Autodesk Fusion 360 part; units mm, degrees
note: some values were not read from the file. Set by a fixed rule: which sketch regions a step uses.
(part 3 of 3)
  line L1807 (17.4645, -45.5732) -> (17.4645, -44.8732)
  line L1808 (18.1645, -45.5732) -> (17.4645, -45.5732)
  line L1809 (18.1645, -44.8732) -> (18.1645, -45.5732)
  line L1810 (17.4645, -47.4132) -> (18.1645, -47.4132)
  line L1811 (17.4645, -48.1132) -> (17.4645, -47.4132)
  line L1812 (18.1645, -48.1132) -> (17.4645, -48.1132)
  line L1813 (18.1645, -47.4132) -> (18.1645, -48.1132)
  line L1814 (17.4645, -49.9532) -> (18.1645, -49.9532)
  line L1815 (17.4645, -50.6532) -> (17.4645, -49.9532)
  line L1816 (18.1645, -50.6532) -> (17.4645, -50.6532)
  line L1817 (18.1645, -49.9532) -> (18.1645, -50.6532)
  line L1818 (51.7545, -37.9058) -> (51.7545, -37.2058)
  line L1819 (51.7545, -37.2058) -> (52.4545, -37.2058)
  line L1820 (52.4545, -37.9058) -> (51.7545, -37.9058)
  line L1821 (52.4545, -37.2058) -> (52.4545, -37.9058)
  line L1822 (51.7545, -40.4458) -> (51.7545, -39.7458)
  line L1823 (51.7545, -39.7458) -> (52.4545, -39.7458)
  line L1824 (52.4545, -40.4458) -> (51.7545, -40.4458)
  line L1825 (52.4545, -39.7458) -> (52.4545, -40.4458)
  line L1826 (51.7545, -42.9858) -> (51.7545, -42.2858)
  line L1827 (51.7545, -42.2858) -> (52.4545, -42.2858)
  line L1828 (52.4545, -42.9858) -> (51.7545, -42.9858)
  line L1829 (52.4545, -42.2858) -> (52.4545, -42.9858)
  line L1830 (51.7545, -45.5258) -> (51.7545, -44.8258)
  line L1831 (51.7545, -44.8258) -> (52.4545, -44.8258)
  line L1832 (52.4545, -45.5258) -> (51.7545, -45.5258)
  line L1833 (52.4545, -44.8258) -> (52.4545, -45.5258)
  line L1834 (51.7545, -48.0658) -> (51.7545, -47.3658)
  line L1835 (51.7545, -47.3658) -> (52.4545, -47.3658)
  line L1836 (52.4545, -48.0658) -> (51.7545, -48.0658)
  line L1837 (52.4545, -47.3658) -> (52.4545, -48.0658)
  line L1838 (51.7545, -50.6058) -> (51.7545, -49.9058)
  line L1839 (51.7545, -49.9058) -> (52.4545, -49.9058)
  line L1840 (52.4545, -50.6058) -> (51.7545, -50.6058)
  line L1841 (52.4545, -49.9058) -> (52.4545, -50.6058)
  line L1842 (11.4445, -17.8682) -> (16.7445, -28.1482)
  line L1843 (11.4445, -28.1482) -> (16.7445, -17.8682)
  line L1844 (18.0945, -17.8682) -> (10.0945, -17.8682)
  line L1845 (10.0945, -17.8682) -> (10.0945, -28.1482)
  line L1846 (10.0945, -28.1482) -> (18.0945, -28.1482)
  line L1847 (18.0945, -28.1482) -> (18.0945, -17.8682)
  line L1848 (18.0945, -17.8682) -> (10.0945, -28.1482) construction
  line L1849 (10.0945, -17.8682) -> (18.0945, -28.1482) construction
  point P0 (62.6345, -26.9982)
  point P1 (68.3345, -18.4982)
  point P2 (5.5845, -52.2482)
  point P3 (68.3345, -52.2482)
  point P4 (4.8345, -21.9982)
  point P5 (52.1045, -35.0158)
  point P6 (17.8145, -31.4432)
  point P7 (17.8145, -40.1432)
  point P8 (14.0945, -23.0082)
  dimension "d3" = 0.7
  dimension "d4" = 0.7
  dimension "d5" = 0.7
  dimension "d6" = 0.7
  dimension "d7" = 0.7
  dimension "d8" = 0.7
  dimension "d11" = 5.08
  dimension "d12" = 0
  dimension "d15" = 10.16
  dimension "d16" = 0
  dimension "d19" = 15.24
  dimension "d20" = 0
  dimension "d21" = 8
  text T0 "+" font "Arial" height 1.3333 align ink ink in box 0 x 0 at (53.2945, -25.6783) x (1, 0) y (0, 1) spacing 1 height is em
  constraint horizontal L1746
  constraint vertical L1747
  constraint horizontal L1748
  constraint vertical L1749
  constraint horizontal L1750
  constraint vertical L1751
  constraint horizontal L1752
  constraint vertical L1753
  constraint horizontal L1754
  constraint vertical L1755
  constraint horizontal L1756
  constraint vertical L1757
  constraint horizontal L1758
  constraint vertical L1759
  constraint horizontal L1760
  constraint vertical L1761
  constraint horizontal L1762
  constraint vertical L1763
  constraint horizontal L1764
  constraint vertical L1765
  constraint horizontal L1766
  constraint vertical L1767
  constraint horizontal L1768
  constraint vertical L1769
  constraint horizontal L1776
  constraint perpendicular L1776 L1777
  constraint parallel L1776 L1778
  constraint parallel L1777 L1779
  constraint coincident L1780 P5
  constraint coincident L1781 P5
  constraint midpoint L1774 P5
  constraint horizontal L1782
  constraint perpendicular L1782 L1783
  constraint parallel L1782 L1784
  constraint parallel L1783 L1785
  constraint coincident L1786 P6
  constraint coincident L1787 P6
  constraint midpoint L1770 P6
  constraint horizontal L1788
  constraint perpendicular L1788 L1789
  constraint parallel L1788 L1790
  constraint parallel L1789 L1791
  constraint coincident L1792 P7
  constraint coincident L1793 P7
  constraint midpoint L1773 P7
  constraint horizontal L1844
  constraint perpendicular L1844 L1845
  constraint parallel L1844 L1846
  constraint parallel L1845 L1847
  constraint coincident L1848 P8
  constraint coincident L1849 P8
  constraint midpoint L1842 P8
  measures "d3" distance of L1777.end L1778.end
  measures "d4" distance of L1776.end L1777.end
  measures "d5" distance of L1783.end L1784.end
  measures "d6" distance of L1782.end L1783.end
  measures "d7" distance of L1789.end L1790.end
  measures "d8" distance of L1788.end L1789.end
  measures "d21" distance of L1845.end L1846.end
extrude "Extrude1" add sketch "Sketch1" sketch "Sketch1" against normal blind 1.6 contours L19 L20 L21 L22 L23 L24 L25 L26 L27 L28 L29 L30 | L70 L71 L74 | L72 L73 L74 | L94 L95 L96 L97 L98 L99 L100 L101 | L102 L103 L104 | L108 L113 L114 L115 L116 L117 L118 L119 L120 L121 | L157 L158 L159 | L155 L156 L159 | L162 L163 L164 | L160 L161 L164 | L169 L174 L175 L176 L177 L178 L179 L180 L181 L182 | L184 L185 L188 | L186 L187 L188 | L196 L197 L198 L199 L200 L201 L202 L203 L204 L205 | L229 L230 L231 L232 L233 L234 L235 L236 L237 L238 | L221 L222 L223 L224 L225 L226 L227 L228 L229 L238 | L246 L247 L248 L249 L250 L251 L252 L253 L254 L255 L256 L257 L258 L259 L260 L261 | L274 L275 L276 L277 L278 L279 L280 L281 L282 L283 | L321 L322 L323 L324 L325 L326 L327 L328 L329 L330 L331 L332 | L349 L350 L351 L352 L353 L354 L355 L356 L357 L358 | L442 L443 L444 L445 L446 L447 L448 L449 L450 L451 L452 L453 | L454 L455 L456 L457 L458 L459 L460 L461 L462 L463 L464 L465 | L521 L522 L523 L524 L525 L526 L527 L528 L529 L530 L531 L532 | L570 L571 L572 L573 L574 L575 L576 L577 L578 L579 L580 L581 | L658 L659 L660 L661 L662 L663 L664 L665 L666 L667 | L650 L651 L652 L653 L654 L655 L656 L657 L658 L667 | L706 L707 L708 | L704 L705 L708 | L716 L717 L718 L719 L720 L721 L722 L723 L724 L725 L726 L727 L728 L729 L730 L731 | L732 L733 L734 L735 L736 L737 L738 L739 L740 L741 L742 L743 L744 L745 L746 L747 | L747 L748 L749 L750 L751 L752 L753 L754 L755 L756 L757 L758 L759 L760 L761 L762 | L780 L781 L782 L783 L784 L785 L786 L787 L788 L789 L1570 L1575 L1576 | L779 L780 L789 L1565 L1566 L1567 L1568 L1569 L1570 | L772 L773 L774 L775 L776 L777 L778 L779 L1565 L1566 L1567 L1568 L1569 L1570 | L781 L782 L1575 L1576 | L791 L792 L1573 L1574 | L791 L792 L1573 | L792 L1573 L1574 | L801 L802 L803 L804 L805 L806 L807 L808 A1 | L801 L802 L803 L804 L805 L806 L807 L808 A1 L1844 | L1654 L1655 L1842 L1843 L1844 | L1652 L1842 L1843 | L1652 L1844 L1845 L1846 | L1653 L1842 L1843 L1846 | L1656 L1842 L1843 | L1656 L1844 L1846 L1847 | L819 L820 L821 L822 L823 L824 L825 L826 L827 L828 L829 L830 | L868 L869 L870 L871 L872 L873 L874 L875 L876 L877 L878 L879 L880 L881 L882 L883 L884 L885 L886 L887 | L926 L927 L928 L929 L930 L931 L932 L933 L934 L935 | L918 L919 L920 L921 L922 L923 L924 L925 L926 L935 | L949 L950 L951 L952 L953 L954 L955 L956 L957 L958 L959 L960 L961 L962 L963 L964 | L1024 L1025 L1026 L1027 L1028 L1029 L1030 L1031 L1032 L1033 L1034 L1035 | L1037 L1038 L1039 L1040 L1041 L1042 L1043 L1044 L1045 L1046 L1047 L1048 L1049 L1050 L1051 L1052 | L1104 L1105 L1106 L1107 L1108 L1109 L1110 L1111 L1112 L1113 | L1096 L1097 L1098 L1099 L1100 L1101 L1102 L1103 L1104 L1113 | L1137 L1138 L1139 L1140 L1141 L1142 L1143 L1144 L1145 L1146 | L1157 L1158 L1159 L1160 L1161 L1162 L1163 L1164 L1165 L1166 L1167 L1168 L1169 L1170 L1171 L1172 L1173 L1174 L1175 L1176 | L1216 L1217 L1218 L1219 L1220 L1221 L1222 L1223 L1224 L1225 L1226 L1227 L1228 L1229 L1230 L1231 | L1233 L1234 L1237 | L1235 L1236 L1237 | L1265 L1266 L1267 L1268 L1269 L1270 L1271 L1272 | L1335 L1336 L1337 L1338 L1339 L1340 L1341 L1342 L1343 L1344 | L1327 L1328 L1329 L1330 L1331 L1332 L1333 L1334 L1335 L1344 | L1360 L1361 L1362 L1363 L1364 L1365 L1366 L1367 L1368 L1369 L1370 L1371 L1372 L1373 L1374 L1375 | L1412 L1413 L1414 L1415 L1416 L1417 L1418 L1419 L1420 L1421 L1422 L1423 L1424 L1425 L1426 L1427 | L1428 L1429 L1430 L1431 L1432 L1433 L1434 L1435 L1436 L1437 L1438 L1439 L1440 L1441 L1442 L1443 L1444 L1445 L1446 L1447 | L1500 L1501 L1502 L1503 L1504 L1505 L1506 L1507 L1508 L1509 L1510 L1511 L1512 L1513 L1514 L1515 | L1522 L1523 L1524 L1525 L1526 L1527 L1528 L1529 L1530 L1531 L1532 L1533 | L1539 L1540 L1541 L1542 L1543 L1544 L1545 L1546 L1547 L1548 L1549 L1550 L1551 L1552 L1553 L1554 | L1596 L1597 L1598 L1599 L1600 L1601 L1602 L1603 L1604 L1605 L1606 L1607 L1608 L1609 L1610 L1611 | L1612 L1613 L1614 L1615 L1616 L1617 L1618 L1619 L1620 L1621 L1622 L1623 L1624 L1625 L1626 L1627 L1628 L1629 L1630 L1631 | L1635 L1636 L1637 L1638 L1642 L1643 L1746 L1747 L1748 L1749 | L1639 L1640 L1641 | L1644 L1645 L1650 L1651 | A0 | L1658 L1761 L1772 L1773 L1789 | L1657 L1758 L1772 L1773 L1789 L1790 L1791 | L1772 L1773 L1789 L1790 L1791 | L1772 L1773 L1789 | L1759 L1772 L1773 L1791 | L1659 L1660 L1661 L1662 L1759 L1760 L1761 | L1660 L1772 L1773 L1788 L1789 L1791 | L1772 L1773 L1791 | L1772 L1773 L1788 L1789 L1791 | L1663 L1664 L1665 L1666 L1685 L1754 L1757 | L1664 L1665 L1666 L1667 L1668 L1669 L1670 L1671 L1672 L1673 L1674 L1675 L1676 L1677 L1678 L1679 L1680 L1681 L1682 L1683 L1684 L1685 L1686 L1687 L1688 L1689 L1690 L1691 L1692 L1693 L1694 L1695 L1696 L1697 L1698 L1699 L1700 L1701 L1702 L1703 L1704 L1705 L1706 L1707 L1708 L1709 L1754 L1755 L1756 L1757 | L1710 L1711 L1712 L1713 | L1714 L1715 L1716 L1717 L1721 L1722 L1750 L1751 L1752 L1753 | L1718 L1719 L1720 | L1725 L1765 L1770 L1771 L1783 | L1724 L1762 L1770 L1771 L1783 L1784 L1785 | L1770 L1771 L1783 L1784 L1785 | L1770 L1771 L1783 | L1763 L1770 L1771 L1785 | L1726 L1727 L1728 L1729 L1763 L1764 L1765 | L1727 L1770 L1771 L1782 L1783 L1785 | L1770 L1771 L1785 | L1770 L1771 L1782 L1783 L1785 | L1731 L1769 L1774 L1775 L1777 | L1730 L1766 L1774 L1775 L1777 L1778 L1779 | L1774 L1775 L1777 L1778 L1779 | L1774 L1775 L1777 | L1767 L1774 L1775 L1779 | L1732 L1733 L1734 L1735 L1767 L1768 L1769 | L1733 L1774 L1775 L1776 L1777 L1779 | L1774 L1775 L1779 | L1774 L1775 L1776 L1777 L1779 | A6 A8 L1737 A9 L1738 L1739 A10 L1740 L1741 | L1794 L1795 L1796 L1797 | L1798 L1799 L1800 L1801 | L1802 L1803 L1804 L1805 | L1806 L1807 L1808 L1809 | L1810 L1811 L1812 L1813 | L1814 L1815 L1816 L1817 | L1818 L1819 L1820 L1821 | L1822 L1823 L1824 L1825 | L1826 L1827 L1828 L1829 | L1830 L1831 L1832 L1833 | L1834 L1835 L1836 L1837 | L1838 L1839 L1840 L1841 of sketch 2 text T0
extrude "Extrude2" add sketch "Sketch1" along normal blind 3.54 contours L1663 L1664 L1665 L1666 L1685 L1754 L1757 | L1664 L1665 L1666 L1667 L1668 L1669 L1670 L1671 L1672 L1673 L1674 L1675 L1676 L1677 L1678 L1679 L1680 L1681 L1682 L1683 L1684 L1685 L1686 L1687 L1688 L1689 L1690 L1691 L1692 L1693 L1694 L1695 L1696 L1697 L1698 L1699 L1700 L1701 L1702 L1703 L1704 L1705 L1706 L1707 L1708 L1709 L1754 L1755 L1756 L1757
sketch "Sketch2" plane through (0, 3.54, 0) normal (0, 1, 0) x (-1, 0, 0)
  line L0 (-24.5845, 51.4982) -> (-45.5845, 51.4982)
  line L1 (-45.5845, 51.4982) -> (-45.5845, 0.4982)
  line L2 (-45.5845, 0.4982) -> (-24.5845, 0.4982)
  line L3 (-24.5845, 0.4982) -> (-24.5845, 51.4982)
  line L4 (-35.0845, 0.4982) -> (-35.0845, -0.8018)
  line L5 (-35.0845, -0.8018) -> (-39.0845, -0.8018)
  line L6 (-39.0845, -0.8018) -> (-31.0845, -0.8018)
  line L7 (-31.0845, -0.8018) -> (-31.0845, 4.7982)
  line L8 (-31.0845, 4.7982) -> (-39.0845, 4.7982)
  line L9 (-39.0845, 4.7982) -> (-39.0845, -0.8018)
  dimension "d24" = 1.3
  dimension "d25" = 4
  dimension "d26" = 8
  dimension "d27" = 5.6
  constraint midpoint L2 L4.start
  constraint perpendicular L2 L4
  constraint perpendicular L4 L5
  constraint horizontal L6
  constraint vertical L7
  constraint horizontal L8
  constraint vertical L9
  measures "d24" distance of L4.start L4.end
  measures "d25" distance of L4.end L5.end
  measures "d26" distance of L5.end L6.end
  measures "d27" distance of L5.end L8.end
extrude "Extrude3" add sketch "Sketch2" along normal blind 3 contours L2 L4 L6 L7 | L2 L7 L8 L9 | L2 L4 L5 L6 L9
extrude "Extrude4" add sketch "Sketch1" along normal blind 7 contours L1635 L1636 L1637 L1638 L1642 L1643 L1746 L1747 L1748 L1749 | L1714 L1715 L1716 L1717 L1721 L1722 L1750 L1751 L1752 L1753
extrude "Extrude5" add sketch "Sketch1" along normal blind 2.54 contours L1658 L1761 L1772 L1773 L1789 | L1657 L1758 L1772 L1773 L1789 L1790 L1791 | L1759 L1772 L1773 L1791 | L1659 L1660 L1661 L1662 L1759 L1760 L1761 | L1660 L1772 L1773 L1788 L1789 L1791 | L1725 L1765 L1770 L1771 L1783 | L1724 L1762 L1770 L1771 L1783 L1784 L1785 | L1763 L1770 L1771 L1785 | L1726 L1727 L1728 L1729 L1763 L1764 L1765 | L1727 L1770 L1771 L1782 L1783 L1785 | L1731 L1769 L1774 L1775 L1777 | L1730 L1766 L1774 L1775 L1777 L1778 L1779 | L1767 L1774 L1775 L1779 | L1732 L1733 L1734 L1735 L1767 L1768 L1769 | L1733 L1774 L1775 L1776 L1777 L1779
extrude "Extrude6" add 15 faces at (17.6978, 0, 31.3265) (17.6978, 0, 33.8665) (17.9312, 0, 36.6399) (17.6978, 0, 40.0265) (17.6978, 0, 42.5665) (17.6978, 0, 45.1065) (17.6978, 0, 47.6465) (17.6978, 0, 50.1865) (51.9878, 0, 34.8991) (51.9878, 0, 37.4391) (52.2212, 0, 40.2124) (52.2212, 0, 42.7524) (52.2212, 0, 45.2924) (52.2212, 0, 47.8324) (52.2212, 0, 50.3724) along direction (0, 1, 0) up to surface end surface through (0, 2.54, 0) normal (0, 1, 0) offset 6
extrude "Extrude7" add sketch "Sketch1" along normal blind 9 contours A0
extrude "Extrude8" add sketch "Sketch1" along normal blind 5 contours L1654 L1655 L1842 L1843 L1844 | L1652 L1842 L1843 | L1652 L1844 L1845 L1846 | L1653 L1842 L1843 L1846 | L1656 L1842 L1843 | L1656 L1844 L1846 L1847
extrude "Extrude9" add sketch "Sketch1" along normal blind 3 contours L1644 L1645 L1650 L1651
extrude "Extrude10" add sketch "Sketch1" along normal blind 25 contours L1710 L1711 L1712 L1713
sketch "Sketch3" plane through (7.2345, 0, 0) normal (-1, 0, 0) x (0, 0, 1)
  line L0 (31.2482, 0) -> (54.7482, 0)
  line L1 (54.7482, 0) -> (54.7482, 25)
  line L2 (54.7482, 25) -> (31.2482, 25)
  line L3 (31.2482, 25) -> (31.2482, 0)
  circle A0 centre (42.9982, 13.25) radius 11.75
  circle A1 centre (42.9982, 13.25) radius 10.75
  line L4 (42.9982, 13.25) -> (42.9982, 0)
  line L5 (35.4982, 13.25) -> (35.4982, 0)
  line L6 (50.4982, 13.25) -> (50.4982, 0)
  line L7 (31.2482, 13.25) -> (54.7482, 13.25)
  dimension "d44" = -1
  dimension "d45" = 7.5
  constraint tangent L2 A0
  constraint tangent L3 A0
  constraint tangent L1 A0
  constraint coincident A0.centre A1.centre
  constraint midpoint L0 L4.end
  constraint symmetric L4 L5.start L6.start
  constraint symmetric L4 L5.end L6.end
  constraint coincident A0 L7.start
  constraint coincident A0 L7.end
  constraint perpendicular L1 L7
extrude "Extrude11" cut sketch "Sketch3" against normal up to surface (6 mm away) contours L0 L3 A0 L5 | L2 L3 A0 | A0 A1 L7 | L1 L2 A0 | L0 L1 A0 L6
sketch "Sketch4" plane through (0, 0, 50.4982) normal (0, 0, 1) x (1, 0, 0)
  line L0 (13.2345, 0) -> (13.2345, 4.205)
  line L1 (13.2345, 4.205) -> (7.2345, 4.205)
  line L2 (7.2345, 4.205) -> (7.2345, 0)
  line L3 (7.2345, 0) -> (13.2345, 0)
  line L4 (13.2345, 4.205) -> (13.2345, 13.25)
  line L5 (13.2345, 13.25) -> (7.2345, 13.25)
  line L6 (7.2345, 13.25) -> (7.2345, 4.205)
  line L7 (7.2345, 4.205) -> (13.2345, 4.205)
  line L8 (13.2345, 13.25) -> (13.2345, 24)
  line L9 (13.2345, 13.25) -> (7.2345, 13.25)
  line L10 (7.2345, 24) -> (7.2345, 13.25)
  line L11 (7.2345, 13.25) -> (13.2345, 13.25)
  line L12 (7.2345, 13.25) -> (8.2345, 13.25)
  line L13 (8.2345, 13.25) -> (8.2345, 24)
  line L14 (13.2345, 13.25) -> (12.2345, 13.25)
  line L15 (12.2345, 13.25) -> (12.2345, 24)
  line L16 (7.2345, 24) -> (13.2345, 24)
  dimension "d48" = 1
  dimension "d49" = 1
  constraint coincident L5.end L6.start
  constraint perpendicular L4 L12
  constraint perpendicular L12 L13
  constraint coincident L4.end L5.start
  constraint coincident L11 L14.end
  constraint perpendicular L14 L15
  constraint coincident L10.start L16.start
  constraint coincident L8.end L16.end
  measures "d48" distance of L5.end L12.end
  measures "d49" distance of L4.end L14.end
extrude "Extrude12" cut sketch "Sketch4" along normal blind 5 and the other way blind 22.5 contours L5 L8 L9 L11 L14 L15 L16 | L5 L9 L10 L11 L12 L13 L16
equation "d11 = 2.54 * 2 mm"
equation "d15 = ( 2.54 * 4 ) * 1 mm"
equation "d19 = ( 2.54 * 6 ) * 1 mm"
equation "d22 = 2.54 mm + 1 mm"
